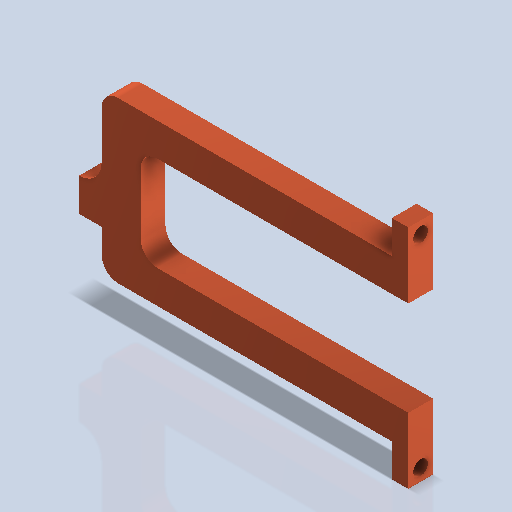
# Autodesk Inventor part: 2
Saved by Autodesk Inventor 2024.2 (Build 282272000, 272)
## iProperties
Created: 2024-05-04
Part Number: 2
Material: Kupfer, Legierung
Document SubType Name: Modeling
Designer: Fabri
Density: 8.92 g/cm^3
Appearance: Kupfer - satiniert
Author: Fabri
Autodesk Inventor part; units mm, degrees
note: some values were not read from the file. Chosen so that the rebuilt part matches the saved one: direction of "Bohrung2".
ref_plane "YZ Plane" through (0, 0, 0) normal (1, 0, 0) x (0, 1, 0)
ref_plane "XZ Plane" through (0, 0, 0) normal (0, 1, 0) x (-1, 0, 0)
ref_plane "XY Plane" through (0, 0, 0) normal (0, 0, 1) x (1, 0, 0)
sketch "Skizze1" plane through (0, 0, 0) normal (0, 1, 0) x (-1, 0, 0)
  line L0 (0, 0) -> (380.5546, 0) construction
  line L1 (20, 97.5) -> (352.5, 97.5)
  line L2 (352.5, -97.5) -> (20, -97.5)
  line L3 (0, 76.1809) -> (0, 137.5)
  line L4 (0, 137.5) -> (20, 137.5)
  line L5 (20, 137.5) -> (20, 97.5)
  line L6 (20, -97.5) -> (20, -137.5)
  line L7 (20, -137.5) -> (0, -137.5)
  line L8 (0, -137.5) -> (0, -73.203)
  line L9 (400, -8.0546) -> (400, -8.0546)
  line L10 (400, -8.0546) -> (400, -48.0546)
  line L11 (400, -48.0546) -> (372.5, -48.0546)
  line L12 (0, 57.5) -> (305, 57.5)
  line L13 (325, 37.5) -> (325, -37.5)
  line L14 (305, -57.5) -> (0, -57.5)
  line L15 (0, -73.203) -> (0, -57.5)
  line L16 (0, 57.5) -> (0, 76.1809)
  line L17 (372.5, 77.5) -> (372.5, 19.4454)
  line L18 (372.5, -48.0546) -> (372.5, -77.5)
  arc A0 (372.5, 19.4454) -> (400, -8.0546) centre (400, 19.4454) ccw
  arc A1 (372.5, 77.5) -> (352.5, 97.5) centre (352.5, 77.5) ccw
  arc A2 (352.5, -97.5) -> (372.5, -77.5) centre (352.5, -77.5) ccw
  arc A3 (325, 37.5) -> (305, 57.5) centre (305, 37.5) ccw
  arc A4 (305, -57.5) -> (325, -37.5) centre (305, -37.5) ccw
  point P0 (372.5, 48.4727)
  dimension "d3" = 57.5
  dimension "d4" = 57.5
  dimension "d7" = 20
  dimension "d8" = 20
  dimension "d11" = 40
  dimension "d12" = 47.5
  dimension "d13" = 27.5
  dimension "d14" = 27.5
  dimension "d18" = 97.5
  dimension "d19" = 97.5
  dimension "d20" = 20
  dimension "d22" = 40
  dimension "d24" = 305
  dimension "d45" = 40
  dimension "d46" = 40
  dimension "d47" = 40
  constraints: 38 end point, 13 perpendicular, 11 point on circle, 10 tangent, 5 centre point, 5 parallel, 4 horizontal, 3 equal radius, 3 vertical alignment, 1 midpoint, 1 vertical
  measures "d3" distance between parallel lines of L14 L0
  measures "d4" distance between parallel lines of L0 L12
  measures "d7" distance between parallel lines of L8 L6
  measures "d8" distance of L3.end L4.end
  measures "d11" distance between parallel lines of L11 L9
  measures "d12" distance between parallel lines of L13 L17
  measures "d13" distance from line of point (372.5, 48.473) L10
  measures "d14" radius of A0
  measures "d18" distance between parallel lines of L0 L1
  measures "d19" distance between parallel lines of L2 L0
  measures "d20" radius of A1
  measures "d22" distance between parallel lines of L2 L14
  measures "d24" distance between parallel lines of L5 L13
  measures "d45" distance between parallel lines of L2 L7
  measures "d46" distance between parallel lines of L4 L1
  measures "d47" distance between parallel lines of L1 L12
extrude "Extrusion1" add sketch "Skizze1" along normal blind 30
sketch "Skizze2" plane through (-400, 0, -48.0546) normal (-1, 0, 0) x (0, 0, 1)
  line L0 (0, 0) -> (0, 30) projected
  line L1 (0, 0) -> (40, 0) projected
  point P0 (48.0546, 0)
  point P1 (24, 15)
  point P2 (0, 15)
  dimension "d34" = 24
  constraints: 1 horizontal alignment, 1 midpoint
  measures "d34" distance from line of L0 point (24, 15)
hole "Bohrung1" at (-400, 15, -24.0546) direction (1, 0, 0) diameter 15.2937 depth 45 thread size "M18x2.5" class "6H" standard "ISO Metric profile"
sketch "Skizze3" plane through (-20, 0, 97.5) normal (-1, 0, 0) x (0, 0, 1)
  line L0 (40, 0) -> (40, 30) projected
  line L1 (-235, 0) -> (-235, 30) projected
  point P0 (-97.5, 0)
  point P1 (25, 15)
  point P2 (-220, 15)
  point P3 (40, 15)
  point P4 (-235, 15)
  dimension "d43" = 15
  dimension "d44" = 15
  constraints: 2 horizontal alignment, 2 midpoint
  measures "d43" distance from line of point (25, 15) L0
  measures "d44" distance from line of L1 point (-220, 15)
hole "Bohrung2" at (-20, 15, 122.5) at (-20, 15, -122.5) direction (1, 0, 0) diameter 18 depth 20
equation "\"d4\" = d3"
equation "\"d8\" = d7"
equation "\"d46\" = d45"
equation "\"d47\" = d22"
